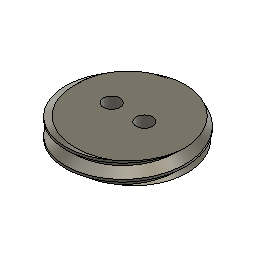
Rosca_KP_v1 (Autodesk Fusion 360 design; units mm, degrees)
part number: 2026-03-20-11-57-37-457
Autodesk Fusion 360 part; units mm, degrees
sketch "Sketch5" plane through (0, 0, 0) normal (0, 1, 0) x (1, 0, 0)
  circle A0 centre (-22, -5) radius 1.5
  circle A1 centre (-28, -5) radius 1.5
  circle A2 centre (-25, -5) radius 10.75
  circle A3 centre (-25, -5) radius 8.75
  point P0 (-25, -5)
  point P1 (-25, -5)
  dimension "d16" = 3
  dimension "d23" = 21.5
  dimension "d24" = 17.5
  constraint coincident P0 A2.centre
  constraint coincident P1 P0
  measures "d16" diameter of A0
  measures "d23" diameter of A2
  measures "d24" diameter of A3
form "Form1" [no effect]
extrude "Extrude4" add sketch "Sketch5" along normal blind 5 contours A2 | A3
thread "Thread1" "ISO Metric profile 22.0 M22x3 M22x3 6g" major diameter 21.7645 minor diameter 18.3374 pitch 3 angle 60 modelled right hand crest width 0.4298 on face at (-14.2634, 3.3333, 5.5358) from (-25, 0, 5) to (-25, 5, 5) crest through (-14.1178, -0.75, 5)
extrude "Extrude1" [rolled back] along distance 5 taper angle 0
